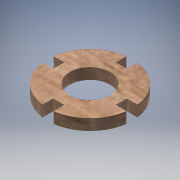
# Autodesk Inventor part: MarkerRing
Saved by Autodesk Inventor 2019 (Build 230136000, 136)
## iProperties
Created: 2019-01-14
Part Number: MarkerRing
Material: Wood (Birch)
Document SubType Name: Modeling
Designer: nxgam
Density: 0.55 g/cm^3
Appearance: Birch - Natural Polished
Author: nxgam
Autodesk Inventor part; units mm, degrees
ref_plane "YZ Plane" through (0, 0, 0) normal (1, 0, 0) x (0, 1, 0)
ref_plane "XZ Plane" through (0, 0, 0) normal (0, 1, 0) x (-1, 0, 0)
ref_plane "XY Plane" through (0, 0, 0) normal (0, 0, 1) x (1, 0, 0)
sketch "Sketch1" plane through (0, 0, 0) normal (0, 1, 0) x (-1, 0, 0)
  circle A0 centre (0, 0) radius 9.271
  arc A1 (19.2643, -2.54) -> (19.2643, 2.54) centre (0, 0) ccw
  line L0 (19.431, 2.54) -> (14.351, 2.54)
  line L1 (14.351, 2.54) -> (14.351, -2.54)
  line L2 (14.351, -2.54) -> (19.431, -2.54)
  line L3 (19.431, -2.54) -> (19.431, 2.54)
  line L4 (19.431, 0) -> (0, 0) construction
  line L5 (-2.54, 19.431) -> (-2.54, 14.351)
  line L6 (-2.54, 14.351) -> (2.54, 14.351)
  line L7 (2.54, 14.351) -> (2.54, 19.431)
  line L8 (2.54, 19.431) -> (-2.54, 19.431)
  line L9 (-19.431, -2.54) -> (-14.351, -2.54)
  line L10 (-14.351, -2.54) -> (-14.351, 2.54)
  line L11 (-14.351, 2.54) -> (-19.431, 2.54)
  line L12 (-19.431, 2.54) -> (-19.431, -2.54)
  line L13 (2.54, -19.431) -> (2.54, -14.351)
  line L14 (2.54, -14.351) -> (-2.54, -14.351)
  line L15 (-2.54, -14.351) -> (-2.54, -19.431)
  line L16 (-2.54, -19.431) -> (2.54, -19.431)
  arc A2 (2.54, -19.2643) -> (13.1001, -14.351) centre (0, 0) ccw
  arc A3 (19.2643, 2.54) -> (2.54, 19.2643) centre (0, 0) ccw
  arc A4 (-19.2643, 2.54) -> (-19.2643, -2.54) centre (0, 0) ccw
  arc A5 (-19.2643, -2.54) -> (-2.54, -19.2643) centre (0, 0) ccw
  arc A6 (2.54, 19.2643) -> (-2.54, 19.2643) centre (0, 0) ccw
  arc A7 (-2.54, 19.2643) -> (-19.2643, 2.54) centre (0, 0) ccw
  arc A8 (13.1001, -14.351) -> (19.2643, -2.54) centre (0, 0) ccw
  arc A9 (-2.54, -19.2643) -> (2.54, -19.2643) centre (0, 0) ccw
  point P0 (0, 19.431)
  point P1 (-19.431, 0)
  point P2 (0, -19.431)
  dimension "d0" = 18.542
  dimension "d1" = 38.862
  dimension "d2" = 5.08
  dimension "d3" = 5.08
  dimension "d6" = 360
  constraints: 34 end point, 18 point on circle, 10 centre point, 9 point on line, 2 coincident, 2 horizontal, 2 parallel, 2 tangent, 1 midpoint, 1 perpendicular, 37 other
  measures "d0" diameter of A0
  measures "d1" diameter of A1
  measures "d2" distance between parallel lines of L2 L0
  measures "d3" distance between parallel lines of L3 L1
extrude "Extrusion1" add sketch "Sketch1" along normal blind 5.08 contours A8 A2 L13 L14 L15 A5 L9 L10 L11 A7 L5 L6 L7 A3 L0 L1 L2
body "Solid1"
